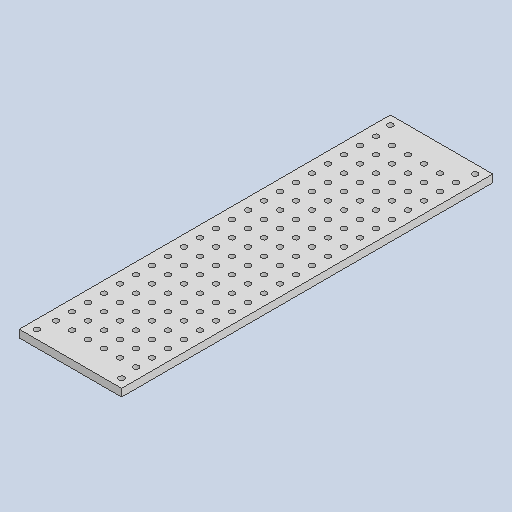
# Autodesk Inventor part: HopperV1
Saved by Autodesk Inventor 2022.1 (Build 261234020, 234B)
## iProperties
Created: 2021-05-28
Part Number: HopperV1
Material: Generic
Document SubType Name: Modeling
Designer: Work
Density: 1 g/cm^3
Appearance: Default
Author: Work
Autodesk Inventor part; units mm, degrees
ref_plane "YZ Plane" through (0, 0, 0) normal (1, 0, 0) x (0, 1, 0)
ref_plane "XZ Plane" through (0, 0, 0) normal (0, 1, 0) x (-1, 0, 0)
ref_plane "XY Plane" through (0, 0, 0) normal (0, 0, 1) x (1, 0, 0)
sketch "Sketch1" plane through (0, 0, 0) normal (0, 1, 0) x (-1, 0, 0)
  line L0 (0, 0) -> (81.28, 0)
  line L1 (81.28, 0) -> (81.28, -294.64)
  line L2 (81.28, -294.64) -> (0, -294.64)
  line L3 (0, -294.64) -> (0, 0)
  dimension "d0" = 81.28
  dimension "d1" = 294.64
  constraints: 8 end point, 3 perpendicular, 1 horizontal
  measures "d0" distance of L0.start L0.end
  measures "d1" distance of L0.end L1.end
extrude "Extrusion1" add sketch "Sketch1" along normal blind 6
sketch "Sketch2" plane through (0, 6, 0) normal (0, 1, 0) x (1, 0, 0)
  circle A0 centre (-7, 7) radius 2.25
  line L0 (-81.28, 0) -> (0, 0) projected
  line L1 (0, 0) -> (0, 294.64) projected
  circle A1 centre (-74.28, 7) radius 2.25
  line L2 (-81.28, 294.64) -> (-81.28, 0) projected
  circle A2 centre (-74.28, 287.64) radius 2.25
  line L3 (0, 294.64) -> (-81.28, 294.64) projected
  circle A3 centre (-7, 287.64) radius 2.25
  dimension "d4" = 4.5
  dimension "d6" = 7
  dimension "d7" = 7
  dimension "d8" = 4.5
  dimension "d9" = 7
  dimension "d10" = 7
  dimension "d11" = 4.5
  dimension "d12" = 7
  dimension "d13" = 7
  dimension "d14" = 4.5
  dimension "d15" = 7
  dimension "d16" = 7
  constraints: 4 centre point
  measures "d4" diameter of A0
  measures "d6" distance from line of L1 A0.centre
  measures "d7" distance from line of L0 A0.centre
  measures "d8" diameter of A1
  measures "d9" distance from line of L2 A1.centre
  measures "d10" distance from line of L0 A1.centre
  measures "d11" diameter of A2
  measures "d12" distance from line of L3 A2.centre
  measures "d13" distance from line of L2 A2.centre
  measures "d14" diameter of A3
  measures "d15" distance from line of L1 A3.centre
  measures "d16" distance from line of L3 A3.centre
extrude "Extrusion2" cut sketch "Sketch2" against normal through all contours A0 | A1 | A2 | A3
sketch "Sketch3" plane through (0, 6, 0) normal (0, 1, 0) x (1, 0, 0)
  circle A0 centre (-8.89, 20.32) radius 2.25
  line L0 (0, 0) -> (0, 294.64) projected
  circle A1 centre (-7, 7) radius 2.25 projected
  line L1 (-81.28, 0) -> (0, 0) projected
  line L2 (0, 0) -> (-4.445, 0)
  dimension "d19" = 4.5
  dimension "d20" = 8.89
  dimension "d64" = 20.32
  constraints: 2 end point, 1 centre point, 1 point on line
  measures "d19" diameter of A0
  measures "d20" distance from line of L0 A0.centre
  measures "d64" distance from line of L1 A0.centre
extrude "Extrusion3" cut sketch "Sketch3" against normal through all contours A0
pattern_linear "Rectangular Pattern1" count 6 spacing 12.7 along (-1, 0, 0) count 21 spacing 12.7 along (0, 0, -1) of "Extrusion3"
body "Solid1"
